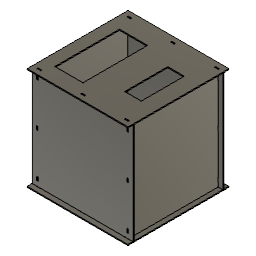
MA GreenForge Greenhouse v21 (Autodesk Fusion 360 design; units mm, degrees)
Autodesk Fusion 360 part; units mm, degrees
sketch "Sketch1" plane through (0, 0, 0) normal (0, 0, 1) x (1, 0, 0)
  line L0 (-377.9, 133.9) -> (-377.9, 137.4)
  line L1 (-631.7, 137.4) -> (-631.7, 133.9)
  line L2 (-631.7, 133.9) -> (-642.2, 133.9)
  line L3 (-642.2, -133.9) -> (-631.7, -133.9)
  line L4 (-367.4, 137.4) -> (-367.4, 133.9)
  line L5 (-642.2, 137.4) -> (-631.7, 137.4)
  line L6 (-657.2, 152.4) -> (-352.4, 152.4)
  line L7 (-352.4, -152.4) -> (-657.2, 152.4) construction
  line L8 (-352.4, 152.4) -> (-352.4, -152.4)
  line L9 (-657.2, -152.4) -> (-657.2, 152.4)
  line L10 (-657.2, -152.4) -> (-352.4, 152.4) construction
  line L11 (-642.2, -137.4) -> (-642.2, -133.9)
  line L12 (-367.4, -137.4) -> (-377.9, -137.4)
  line L13 (-352.4, -152.4) -> (-657.2, -152.4)
  line L14 (-377.9, -133.9) -> (-367.4, -133.9)
  line L15 (-631.7, -137.4) -> (-642.2, -137.4)
  line L16 (-377.9, -137.4) -> (-377.9, -133.9)
  line L17 (-367.4, -133.9) -> (-367.4, -137.4)
  line L18 (-631.7, -133.9) -> (-631.7, -137.4)
  line L19 (-642.2, 133.9) -> (-642.2, 137.4)
  line L20 (-377.9, 137.4) -> (-367.4, 137.4)
  line L21 (-367.4, 133.9) -> (-377.9, 133.9)
  line L22 (-499.55, 133.9) -> (-510.05, 133.9)
  line L23 (-510.05, 133.9) -> (-510.05, 137.4)
  line L24 (-510.05, 137.4) -> (-499.55, 137.4)
  line L25 (-499.55, 137.4) -> (-499.55, 133.9)
  line L26 (-499.55, 133.9) -> (-510.05, 137.4) construction
  line L27 (-510.05, 133.9) -> (-499.55, 137.4) construction
  line L28 (-499.55, -137.4) -> (-510.05, -137.4)
  line L29 (-510.05, -137.4) -> (-510.05, -133.9)
  line L30 (-510.05, -133.9) -> (-499.55, -133.9)
  line L31 (-499.55, -133.9) -> (-499.55, -137.4)
  line L32 (-499.55, -137.4) -> (-510.05, -133.9) construction
  line L33 (-510.05, -137.4) -> (-499.55, -133.9) construction
  line L34 (-126.9, 137.4) -> (-126.9, 133.9)
  line L35 (126.9, 133.9) -> (126.9, 137.4)
  line L36 (-137.4, 133.9) -> (-137.4, 137.4)
  line L37 (137.4, -133.9) -> (137.4, -137.4)
  line L38 (-5.25, 137.4) -> (5.25, 137.4)
  line L39 (5.25, -137.4) -> (-5.25, -137.4)
  line L40 (152.4, 152.4) -> (152.4, -152.4)
  line L41 (126.9, -137.4) -> (126.9, -133.9)
  line L42 (-152.4, -152.4) -> (-152.4, 152.4)
  line L43 (-5.25, -133.9) -> (5.25, -133.9)
  line L44 (-5.25, 133.9) -> (-5.25, 137.4)
  line L45 (-5.25, 133.9) -> (5.25, 137.4) construction
  line L46 (-137.4, 137.4) -> (-126.9, 137.4)
  line L47 (5.25, 133.9) -> (-5.25, 133.9)
  line L48 (126.9, 137.4) -> (137.4, 137.4)
  line L49 (152.4, -152.4) -> (-152.4, 152.4) construction
  line L50 (5.25, 133.9) -> (-5.25, 137.4) construction
  line L51 (-5.25, -137.4) -> (-5.25, -133.9)
  line L52 (-126.9, -133.9) -> (-126.9, -137.4)
  line L53 (137.4, 133.9) -> (126.9, 133.9)
  line L54 (152.4, -152.4) -> (-152.4, -152.4)
  line L55 (5.25, -137.4) -> (-5.25, -133.9) construction
  line L56 (5.25, -133.9) -> (5.25, -137.4)
  line L57 (137.4, -137.4) -> (126.9, -137.4)
  line L58 (5.25, 137.4) -> (5.25, 133.9)
  line L59 (126.9, -133.9) -> (137.4, -133.9)
  line L60 (-152.4, 152.4) -> (152.4, 152.4)
  line L61 (-152.4, -152.4) -> (152.4, 152.4) construction
  line L62 (-5.25, -137.4) -> (5.25, -133.9) construction
  line L63 (-126.9, 133.9) -> (-137.4, 133.9)
  line L64 (-126.9, -137.4) -> (-137.4, -137.4)
  line L65 (137.4, 137.4) -> (137.4, 133.9)
  line L66 (-137.4, -133.9) -> (-126.9, -133.9)
  line L67 (-137.4, -137.4) -> (-137.4, -133.9)
  line L68 (137.4, 349.4) -> (127.4, 352.4) construction
  line L69 (137.4, 352.4) -> (137.4, 349.4)
  line L70 (4.75, 352.4) -> (127.4, 352.4)
  line L71 (-5.25, 349.4) -> (4.75, 352.4) construction
  line L72 (-137.4, 349.4) -> (-137.4, 352.4)
  line L73 (-5.25, 349.4) -> (-5.25, 352.4)
  line L74 (-152.4, 352.4) -> (-137.4, 352.4)
  line L75 (-137.4, 349.4) -> (-127.4, 352.4) construction
  line L76 (-127.4, 349.4) -> (-137.4, 352.4) construction
  line L77 (137.4, 352.4) -> (152.4, 352.4)
  line L78 (127.4, 349.4) -> (127.4, 352.4)
  line L79 (127.4, 349.4) -> (137.4, 352.4) construction
  line L80 (4.75, 349.4) -> (-5.25, 352.4) construction
  line L81 (137.4, 349.4) -> (127.4, 349.4)
  line L82 (152.4, 352.4) -> (152.4, 621.2)
  line L83 (-127.4, 352.4) -> (-5.25, 352.4)
  line L84 (4.75, 352.4) -> (4.75, 349.4)
  line L85 (-5.25, 621.2) -> (4.75, 624.2) construction
  line L86 (4.75, 621.2) -> (-5.25, 624.2) construction
  line L87 (127.4006, 621.2) -> (127.4006, 624.2)
  line L88 (127.4006, 624.2) -> (137.4, 624.3068)
  line L89 (137.4, 624.3068) -> (137.4, 621.2)
  line L90 (-137.4, 621.2) -> (-152.4, 621.2)
  line L91 (-5.25, 624.2) -> (4.75, 624.2)
  line L92 (-127.4, 624.2) -> (-127.4, 621.2)
  line L93 (-5.25, 621.2) -> (-5.25, 624.2)
  line L94 (4.75, 624.2) -> (4.75, 621.2)
  line L95 (-137.4, 621.2) -> (-127.4, 624.2) construction
  line L96 (-137.4, 624.2) -> (-127.4, 624.2)
  line L97 (152.4, 621.2) -> (137.4, 621.2)
  line L98 (-5.25, 621.2) -> (-127.4, 621.2)
  line L99 (127.4006, 621.2) -> (4.75, 621.2)
  line L100 (-127.4, 621.2) -> (-137.4, 624.2) construction
  line L101 (-137.4, 621.2) -> (-137.4, 624.2)
  line L102 (-152.4, 621.2) -> (152.4, 352.4) construction
  line L103 (-152.4, 621.2) -> (-152.4, 352.4)
  line L104 (4.75, 349.4) -> (-5.25, 349.4)
  line L105 (-127.4, 349.4) -> (-137.4, 349.4)
  line L106 (127.4006, 621.2) -> (137.4, 624.3068) construction
  line L107 (137.4, 621.2) -> (127.4006, 624.2) construction
  line L108 (152.4, 621.2) -> (-152.4, 352.4) construction
  line L109 (-127.4, 352.4) -> (-127.4, 349.4)
  line L110 (-620.875, 90) -> (-535.875, 90)
  line L111 (-535.875, 90) -> (-535.875, -105)
  line L112 (-535.875, -105) -> (-620.875, -105)
  line L113 (-620.875, -105) -> (-620.875, 90)
  line L114 (-400, 65) -> (-450, 65)
  line L115 (-450, 65) -> (-450, -65)
  line L116 (-450, -65) -> (-400, -65)
  line L117 (-400, -65) -> (-400, 65)
  line L118 (-458.1406, 349.4) -> (-468.1406, 349.4)
  line L119 (-335.4884, 624.2) -> (-325.4906, 623.9923)
  line L120 (-468.1406, 624.2) -> (-468.1406, 621.2)
  line L121 (-325.4906, 352.4) -> (-310.4906, 352.4)
  line L122 (-615.2906, 621.2) -> (-310.4906, 352.4) construction
  line L123 (-335.4906, 349.4) -> (-325.4906, 352.4) construction
  line L124 (-458.1406, 352.4) -> (-335.4906, 352.4)
  line L125 (-458.1406, 621.2) -> (-458.1406, 624.2)
  line L126 (-310.4906, 621.2) -> (-615.2906, 352.4) construction
  line L127 (-325.4906, 349.4) -> (-335.4906, 349.4)
  line L128 (-335.4884, 621.2) -> (-458.1406, 621.2)
  line L129 (-600.2906, 621.2) -> (-600.2906, 624.2)
  line L130 (-468.1406, 349.4) -> (-468.1406, 352.4)
  line L131 (-335.4884, 621.2) -> (-325.4906, 623.9923) construction
  line L132 (-615.2906, 352.4) -> (-600.2906, 352.4)
  line L133 (-590.2906, 352.4) -> (-468.1406, 352.4)
  line L134 (-590.2906, 624.2) -> (-590.2906, 621.2)
  line L135 (-600.2906, 349.4) -> (-590.2906, 352.4) construction
  line L136 (-590.2906, 621.2) -> (-600.2906, 624.2) construction
  line L137 (-590.2906, 349.4) -> (-600.2906, 352.4) construction
  line L138 (-468.1406, 621.2) -> (-590.2906, 621.2)
  line L139 (-590.2906, 352.4) -> (-590.2906, 349.4)
  line L140 (-600.2906, 349.4) -> (-600.2906, 352.4)
  line L141 (-325.4906, 623.9923) -> (-325.4906, 621.2)
  line L142 (-335.4884, 621.2) -> (-335.4884, 624.2)
  line L143 (-458.1406, 352.4) -> (-458.1406, 349.4)
  line L144 (-335.4906, 349.4) -> (-335.4906, 352.4)
  line L145 (-458.1406, 621.2) -> (-468.1406, 624.2) construction
  line L146 (-600.2906, 621.2) -> (-615.2906, 621.2)
  line L147 (-600.2906, 624.2) -> (-590.2906, 624.2)
  line L148 (-590.2906, 349.4) -> (-600.2906, 349.4)
  line L149 (-615.2906, 621.2) -> (-615.2906, 352.4)
  line L150 (-600.2906, 621.2) -> (-590.2906, 624.2) construction
  line L151 (-458.1406, 624.2) -> (-468.1406, 624.2)
  line L152 (-468.1406, 349.4) -> (-458.1406, 352.4) construction
  line L153 (-310.4906, 352.4) -> (-310.4906, 621.2)
  line L154 (-310.4906, 621.2) -> (-325.4906, 621.2)
  line L155 (-325.4906, 621.2) -> (-335.4884, 624.2) construction
  line L156 (-458.1406, 349.4) -> (-468.1406, 352.4) construction
  line L157 (-325.4906, 349.4) -> (-335.4906, 352.4) construction
  line L158 (-325.4906, 352.4) -> (-325.4906, 349.4)
  line L159 (-468.1406, 621.2) -> (-458.1406, 624.2) construction
  line L160 (377.4, -147.708) -> (377.4, -150.708)
  line L161 (632.2, 160.092) -> (642.2, 160.092)
  line L162 (367.4, 157.092) -> (377.4, 160.092) construction
  line L163 (632.2, 157.092) -> (632.2, 160.092)
  line L164 (499.55, 160.092) -> (509.55, 160.092)
  line L165 (642.2, 160.092) -> (642.2, 157.092)
  line L166 (499.55, 157.092) -> (499.55, 160.092)
  line L167 (509.55, 160.092) -> (509.55, 157.092)
  line L168 (367.4, 157.092) -> (352.4, 157.092)
  line L169 (501.587, -147.708) -> (632.2, -147.708)
  line L170 (367.4, 157.092) -> (367.4, 160.092)
  line L171 (499.55, 157.092) -> (377.4, 157.092)
  line L172 (367.4, 160.092) -> (377.4, 160.092)
  line L173 (377.4, 160.092) -> (377.4, 157.092)
  line L174 (632.2, 157.092) -> (642.2, 160.092) construction
  line L175 (642.2, 157.092) -> (632.2, 160.092) construction
  line L176 (352.4, -147.708) -> (367.4, -147.708)
  line L177 (642.2, -147.708) -> (642.2, -150.708)
  line L178 (367.4, -150.708) -> (377.4, -147.708) construction
  line L179 (642.2, -150.708) -> (632.2, -150.708)
  line L180 (509.55, -148.7712) -> (499.55, -148.7712)
  line L181 (509.55, -143.5517) -> (509.55, -148.7712)
  line L182 (499.55, -148.7712) -> (509.55, -143.5517) construction
  line L183 (632.2, -150.708) -> (642.2, -147.708) construction
  line L184 (642.2, -150.708) -> (632.2, -147.708) construction
  line L185 (377.4, -150.708) -> (367.4, -150.708)
  line L186 (632.2, -150.708) -> (632.2, -147.708)
  line L187 (509.55, -148.7712) -> (499.55, -145.7712) construction
  line L188 (642.2, -147.708) -> (657.2, -147.708)
  line L189 (377.4, -147.708) -> (506.006, -147.708)
  line L190 (499.55, -148.7712) -> (499.55, -145.7712)
  line L191 (657.2, 157.092) -> (352.4, -147.708) construction
  line L192 (377.4, -150.708) -> (367.4, -147.708) construction
  line L193 (367.4, -150.708) -> (367.4, -147.708)
  line L194 (657.2, -147.708) -> (657.2, 157.092)
  line L195 (499.55, 157.092) -> (509.55, 160.092) construction
  line L196 (377.4, 157.092) -> (367.4, 160.092) construction
  line L197 (509.55, 157.092) -> (499.55, 160.092) construction
  line L198 (657.2, 157.092) -> (642.2, 157.092)
  line L199 (632.2, 157.092) -> (509.55, 157.092)
  line L200 (352.4, 157.092) -> (657.2, -147.708) construction
  line L201 (352.4, 157.092) -> (352.4, -147.708)
  line L202 (370.9, -132.708) -> (367.4, -132.708)
  line L203 (367.4, -132.708) -> (367.4, -122.208)
  line L204 (367.4, -122.208) -> (370.9, -122.208)
  line L205 (370.9, -122.208) -> (370.9, -132.708)
  line L206 (370.9, -132.708) -> (367.4, -122.208) construction
  line L207 (367.4, -132.708) -> (370.9, -122.208) construction
  line L208 (369.15, -0.558) -> (365.65, -0.558)
  line L209 (365.65, -0.558) -> (365.65, 9.942)
  line L210 (365.65, 9.942) -> (369.15, 9.942)
  line L211 (369.15, 9.942) -> (369.15, -0.558)
  line L212 (369.15, -0.558) -> (365.65, 9.942) construction
  line L213 (365.65, -0.558) -> (369.15, 9.942) construction
  line L214 (370.9, 131.592) -> (367.4, 131.592)
  line L215 (367.4, 131.592) -> (367.4, 142.092)
  line L216 (367.4, 142.092) -> (370.9, 142.092)
  line L217 (370.9, 142.092) -> (370.9, 131.592)
  line L218 (370.9, 131.592) -> (367.4, 142.092) construction
  line L219 (367.4, 131.592) -> (370.9, 142.092) construction
  line L220 (638.7, 131.592) -> (642.2, 131.592)
  line L221 (642.2, 131.592) -> (642.2, 142.092)
  line L222 (642.2, 142.092) -> (638.7, 142.092)
  line L223 (638.7, 142.092) -> (638.7, 131.592)
  line L224 (638.7, 131.592) -> (642.2, 142.092) construction
  line L225 (642.2, 131.592) -> (638.7, 142.092) construction
  line L226 (638.7, -0.558) -> (642.2, -0.558)
  line L227 (642.2, -0.558) -> (642.2, 9.942)
  line L228 (642.2, 9.942) -> (638.7, 9.942)
  line L229 (638.7, 9.942) -> (638.7, -0.558)
  line L230 (638.7, -0.558) -> (642.2, 9.942) construction
  line L231 (642.2, -0.558) -> (638.7, 9.942) construction
  line L232 (642.2, -132.708) -> (638.7, -132.708)
  line L233 (638.7, -132.708) -> (638.7, -122.208)
  line L234 (638.7, -122.208) -> (642.2, -122.208)
  line L235 (642.2, -122.208) -> (642.2, -132.708)
  line L236 (642.2, -132.708) -> (638.7, -122.208) construction
  line L237 (638.7, -132.708) -> (642.2, -122.208) construction
  line L238 (657.2, 661.892) -> (642.2, 661.892)
  line L239 (638.7, 504.242) -> (642.2, 504.242)
  line L240 (367.4, 661.892) -> (377.4, 664.892) construction
  line L241 (642.2, 372.092) -> (638.7, 382.592) construction
  line L242 (365.65, 514.742) -> (369.15, 514.742)
  line L243 (370.9, 636.392) -> (367.4, 646.892) construction
  line L244 (632.2, 354.092) -> (632.2, 357.092)
  line L245 (499.55, 661.892) -> (509.55, 664.892) construction
  line L246 (370.9, 636.392) -> (367.4, 636.392)
  line L247 (499.55, 661.892) -> (377.4, 661.892)
  line L248 (367.4, 661.892) -> (352.4, 661.892)
  line L249 (642.2, 636.392) -> (642.2, 646.892)
  line L250 (377.4, 664.892) -> (377.4, 661.892)
  line L251 (638.7, 372.092) -> (638.7, 382.592)
  line L252 (642.2, 354.092) -> (632.2, 357.092) construction
  line L253 (367.4, 636.392) -> (370.9, 646.892) construction
  line L254 (509.55, 357.092) -> (509.55, 354.092)
  line L255 (499.55, 354.092) -> (499.55, 357.092)
  line L256 (370.9, 646.892) -> (370.9, 636.392)
  line L257 (369.15, 504.242) -> (365.65, 504.242)
  line L258 (638.7, 372.092) -> (642.2, 382.592) construction
  line L259 (377.4, 661.892) -> (367.4, 664.892) construction
  line L260 (367.4, 372.092) -> (367.4, 382.592)
  line L261 (642.2, 357.092) -> (642.2, 354.092)
  line L262 (367.4, 661.892) -> (367.4, 664.892)
  line L263 (642.2, 382.592) -> (642.2, 372.092)
  line L264 (377.4, 354.092) -> (367.4, 357.092) construction
  line L265 (509.55, 354.092) -> (499.55, 357.092) construction
  line L266 (367.4, 354.092) -> (377.4, 357.092) construction
  line L267 (499.55, 354.092) -> (509.55, 357.092) construction
  line L268 (632.2, 354.092) -> (642.2, 357.092) construction
  line L269 (367.4, 646.892) -> (370.9, 646.892)
  line L270 (377.4, 357.092) -> (377.4, 354.092)
  line L271 (370.9, 372.092) -> (367.4, 382.592) construction
  line L272 (509.55, 354.092) -> (499.55, 354.092)
  line L273 (509.55, 357.092) -> (632.2, 357.092)
  line L274 (370.9, 382.592) -> (370.9, 372.092)
  line L275 (642.2, 354.092) -> (632.2, 354.092)
  line L276 (642.2, 664.892) -> (642.2, 661.892)
  line L277 (632.2, 661.892) -> (642.2, 664.892) construction
  line L278 (367.4, 354.092) -> (367.4, 357.092)
  line L279 (370.9, 372.092) -> (367.4, 372.092)
  line L280 (632.2, 661.892) -> (509.55, 661.892)
  line L281 (377.4, 354.092) -> (367.4, 354.092)
  line L282 (367.4, 382.592) -> (370.9, 382.592)
  line L283 (352.4, 357.092) -> (367.4, 357.092)
  line L284 (367.4, 372.092) -> (370.9, 382.592) construction
  line L285 (657.2, 661.892) -> (352.4, 357.092) construction
  line L286 (638.7, 636.392) -> (642.2, 636.392)
  line L287 (499.55, 664.892) -> (509.55, 664.892)
  line L288 (642.2, 636.392) -> (638.7, 646.892) construction
  line L289 (509.55, 661.892) -> (499.55, 664.892) construction
  line L290 (642.2, 514.742) -> (638.7, 514.742)
  line L291 (365.65, 504.242) -> (365.65, 514.742)
  line L292 (352.4, 661.892) -> (352.4, 357.092)
  line L293 (369.15, 514.742) -> (369.15, 504.242)
  line L294 (352.4, 661.892) -> (657.2, 357.092) construction
  line L295 (632.2, 664.892) -> (642.2, 664.892)
  line L296 (499.55, 661.892) -> (499.55, 664.892)
  line L297 (642.2, 646.892) -> (638.7, 646.892)
  line L298 (632.2, 661.892) -> (632.2, 664.892)
  line L299 (638.7, 636.392) -> (642.2, 646.892) construction
  line L300 (367.4, 636.392) -> (367.4, 646.892)
  line L301 (367.4, 664.892) -> (377.4, 664.892)
  line L302 (642.2, 661.892) -> (632.2, 664.892) construction
  line L303 (638.7, 382.592) -> (642.2, 382.592)
  line L304 (642.2, 357.092) -> (657.2, 357.092)
  line L305 (377.4, 357.092) -> (499.55, 357.092)
  line L306 (642.2, 372.092) -> (638.7, 372.092)
  line L307 (642.2, 504.242) -> (638.7, 514.742) construction
  line L308 (369.15, 504.242) -> (365.65, 514.742) construction
  line L309 (657.2, 357.092) -> (657.2, 661.892)
  line L310 (638.7, 514.742) -> (638.7, 504.242)
  line L311 (638.7, 504.242) -> (642.2, 514.742) construction
  line L312 (642.2, 504.242) -> (642.2, 514.742)
  line L313 (638.7, 646.892) -> (638.7, 636.392)
  line L314 (509.55, 664.892) -> (509.55, 661.892)
  line L315 (365.65, 504.242) -> (369.15, 514.742) construction
  point P0 (-504.8, 0)
  point P1 (-504.8, 135.65)
  point P2 (-504.8, -135.65)
  point P3 (0, 135.65)
  point P4 (0, -135.65)
  point P5 (-132.4, 622.7)
  point P6 (-0.25, 622.7)
  point P7 (0, 486.8)
  point P8 (-132.4, 350.9)
  point P9 (132.4, 350.9)
  point P10 (132.3129, 622.7262)
  point P11 (-595.2906, 350.9)
  point P12 (-330.4906, 350.9)
  point P13 (-595.2906, 622.7)
  point P14 (-463.1406, 622.7)
  point P15 (-330.3102, 622.6462)
  point P16 (-462.8906, 486.8)
  point P17 (372.4, -149.208)
  point P18 (504.8, 4.692)
  point P19 (372.4, 158.592)
  point P20 (504.55, 158.592)
  point P21 (637.2, -149.208)
  point P22 (637.2, 158.592)
  point P23 (369.15, -127.458)
  point P24 (367.4, 4.692)
  point P25 (369.15, 136.842)
  point P26 (640.45, 136.842)
  point P27 (640.45, 4.692)
  point P28 (640.45, -127.458)
  point P29 (640.45, 509.492)
  point P30 (640.45, 641.642)
  point P31 (367.4, 509.492)
  point P32 (640.45, 377.342)
  point P33 (369.15, 377.342)
  point P34 (372.4, 355.592)
  point P35 (504.8, 509.492)
  point P36 (372.4, 663.392)
  point P37 (504.55, 663.392)
  point P38 (637.2, 355.592)
  point P39 (637.2, 663.392)
  point P40 (369.15, 641.642)
  dimension "d45" = 304.8
  dimension "d46" = 304.8
  dimension "d47" = 10.5
  dimension "d48" = 3.5
  dimension "d49" = 15
  dimension "d50" = 15
  dimension "d51" = 15
  dimension "d52" = 15
  dimension "d53" = 3.5
  dimension "d54" = 15
  dimension "d55" = 15
  dimension "d56" = 15
  dimension "d57" = 15
  dimension "d96" = 147.15
  dimension "d97" = 15
  dimension "d99" = 147.15
  dimension "d100" = 304.8
  dimension "d101" = 304.8
  dimension "d102" = 10.5
  dimension "d103" = 3.5
  dimension "d104" = 15
  dimension "d105" = 15
  dimension "d106" = 15
  dimension "d107" = 15
  dimension "d108" = 3.5
  dimension "d109" = 15
  dimension "d110" = 15
  dimension "d111" = 15
  dimension "d112" = 15
  dimension "d113" = 147.15
  dimension "d114" = 15
  dimension "d116" = 147.15
  dimension "d117" = 200
  dimension "d163" = 15
  dimension "d164" = 15
  dimension "d260" = 268.8
  dimension "d261" = 304.8
  dimension "d262" = 10
  dimension "d263" = 3
  dimension "d264" = 15
  dimension "d265" = 10
  dimension "d266" = 10
  dimension "d267" = 15
  dimension "d268" = 15
  dimension "d269" = 15
  dimension "d281" = 147.15
  dimension "d282" = 147.15
  dimension "d286" = 200
  dimension "d336" = 85
  dimension "d337" = 195
  dimension "d338" = 31.075
  dimension "d340" = 47.6
  dimension "d341" = 130
  dimension "d342" = 87.4
  dimension "d343" = 50
  dimension "d356" = 3
  dimension "d357" = 90
  dimension "d358" = 3
  dimension "d359" = 268.8
  dimension "d360" = 304.8
  dimension "d361" = 10
  dimension "d362" = 3
  dimension "d363" = 15
  dimension "d364" = 10
  dimension "d365" = 10
  dimension "d366" = 15
  dimension "d367" = 15
  dimension "d368" = 15
  dimension "d370" = 147.15
  dimension "d371" = 3
  dimension "d372" = 90
  dimension "d373" = 3
  dimension "d374" = 304.8
  dimension "d375" = 304.8
  dimension "d376" = 10
  dimension "d377" = 3
  dimension "d378" = 15
  dimension "d379" = 10
  dimension "d380" = 10
  dimension "d381" = 15
  dimension "d382" = 15
  dimension "d383" = 15
  dimension "d390" = 147.15
  dimension "d391" = 147.15
  dimension "d410" = 200
  dimension "d429" = 15
  dimension "d430" = 15
  dimension "d431" = 3.5
  dimension "d432" = 10.5
  dimension "d433" = 15
  dimension "d434" = 147.15
  dimension "d435" = 15
  dimension "d436" = 15
  dimension "d437" = 15
  dimension "d438" = 15
  dimension "d439" = 3.5
  dimension "d440" = 15
  dimension "d441" = 15
  dimension "d442" = 15
  dimension "d443" = 147.15
  dimension "d473" = 304.8
  dimension "d474" = 304.8
  dimension "d475" = 10
  dimension "d476" = 3
  dimension "d477" = 15
  dimension "d478" = 10
  dimension "d479" = 10
  dimension "d480" = 15
  dimension "d481" = 15
  dimension "d482" = 15
  dimension "d483" = 147.15
  dimension "d484" = 147.15
  dimension "d485" = 15
  dimension "d486" = 15
  dimension "d487" = 3.5
  dimension "d488" = 10.5
  dimension "d489" = 15
  dimension "d490" = 147.15
  dimension "d491" = 15
  dimension "d492" = 15
  dimension "d493" = 15
  dimension "d494" = 15
  dimension "d495" = 3.5
  dimension "d496" = 15
  dimension "d497" = 15
  dimension "d498" = 15
  dimension "d499" = 147.15
  dimension "d500" = 200
  dimension "d501" = 200
  dimension "d522" = 147.15
  dimension "d535" = 3
  dimension "d537" = 90
  dimension "d538" = 90
  dimension "d539" = 90
  dimension "d540" = 90
  dimension "d541" = 90
  constraint horizontal L13
  constraint perpendicular L9 L13
  constraint parallel L6 L13
  constraint parallel L8 L9
  constraint coincident P0 L7
  constraint coincident P0 L10
  constraint horizontal L5
  constraint vertical L1
  constraint horizontal L2
  constraint vertical L19
  constraint horizontal L20
  constraint vertical L4
  constraint horizontal L21
  constraint vertical L0
  constraint horizontal L3
  constraint vertical L18
  constraint horizontal L15
  constraint vertical L11
  constraint horizontal L14
  constraint vertical L17
  constraint horizontal L12
  constraint vertical L16
  constraint equal L2 L20
  constraint equal L2 L3
  constraint equal L3 L14
  constraint equal L0 L1
  constraint equal L16 L18
  constraint horizontal L22
  constraint perpendicular L22 L23
  constraint parallel L22 L24
  constraint parallel L23 L25
  constraint coincident L26 P1
  constraint coincident L27 P1
  constraint equal L19 L23
  constraint equal L5 L24
  constraint horizontal L28
  constraint perpendicular L28 L29
  constraint parallel L28 L30
  constraint parallel L29 L31
  constraint coincident L32 P2
  constraint coincident L33 P2
  constraint equal L11 L29
  constraint equal L3 L30
  constraint horizontal L54
  constraint perpendicular L42 L54
  constraint parallel L54 L60
  constraint parallel L40 L42
  constraint coincident origin L49
  constraint coincident origin L61
  constraint horizontal L46
  constraint vertical L34
  constraint horizontal L63
  constraint vertical L36
  constraint horizontal L48
  constraint vertical L65
  constraint horizontal L53
  constraint vertical L35
  constraint horizontal L66
  constraint vertical L52
  constraint horizontal L64
  constraint vertical L67
  constraint horizontal L59
  constraint vertical L37
  constraint horizontal L57
  constraint vertical L41
  constraint equal L48 L63
  constraint equal L63 L66
  constraint equal L59 L66
  constraint equal L34 L35
  constraint equal L41 L52
  constraint horizontal L47
  constraint perpendicular L44 L47
  constraint parallel L38 L47
  constraint parallel L44 L58
  constraint coincident P3 L50
  constraint coincident P3 L45
  constraint equal L36 L44
  constraint equal L38 L46
  constraint horizontal L39
  constraint perpendicular L39 L51
  constraint parallel L39 L43
  constraint parallel L51 L56
  constraint coincident P4 L55
  constraint coincident P4 L62
  constraint equal L51 L67
  constraint equal L43 L66
  constraint collinear L6 L60
  constraint horizontal L97
  constraint perpendicular L97 L103
  constraint parallel L74 L97
  constraint parallel L82 L103
  constraint coincident P7 L108
  constraint coincident P7 L102
  constraint parallel L92 L101
  constraint coincident P5 L100
  constraint coincident P5 L95
  constraint parallel L87 L89
  constraint coincident P10 L107
  constraint coincident P10 L106
  constraint horizontal L105
  constraint perpendicular L72 L105
  constraint parallel L72 L109
  constraint coincident P8 L76
  constraint coincident P8 L75
  constraint horizontal L81
  constraint perpendicular L78 L81
  constraint parallel L69 L78
  constraint coincident P9 L68
  constraint coincident P9 L79
  constraint equal L72 L78
  constraint equal L78 L87
  constraint equal L87 L101
  constraint equal L88 L96
  constraint collinear L90 L97
  constraint collinear L97 L99
  constraint collinear L74 L83
  constraint collinear L77 L83
  constraint parallel L93 L94
  constraint coincident P6 L86
  constraint coincident P6 L85
  constraint equal L92 L93
  constraint equal L91 L96
  constraint horizontal L104
  constraint perpendicular L73 L104
  constraint parallel L73 L84
  constraint equal L72 L73
  constraint equal L104 L105
  constraint coincident L73.end L80
  constraint coincident L70.start L71
  constraint collinear L70 L83
  constraint collinear L98 L99
  constraint collinear L40 L82
  constraint horizontal L110
  constraint vertical L111
  constraint horizontal L112
  constraint vertical L113
  constraint horizontal L114
  constraint vertical L115
  constraint horizontal L116
  constraint vertical L117
  constraint coincident L73.end L80.end
  constraint horizontal L154
  constraint perpendicular L149 L154
  constraint parallel L132 L154
  constraint parallel L149 L153
  constraint coincident P16 L126
  constraint coincident P16 L122
  constraint parallel L129 L134
  constraint coincident P13 L136
  constraint coincident P13 L150
  constraint parallel L141 L142
  constraint coincident P15 L155
  constraint coincident P15 L131
  constraint horizontal L148
  constraint perpendicular L140 L148
  constraint parallel L139 L140
  constraint coincident P11 L137
  constraint coincident P11 L135
  constraint horizontal L127
  constraint perpendicular L127 L144
  constraint parallel L144 L158
  constraint coincident P12 L157
  constraint coincident P12 L123
  constraint equal L140 L144
  constraint equal L142 L144
  constraint equal L129 L142
  constraint equal L119 L147
  constraint collinear L146 L154
  constraint collinear L128 L154
  constraint collinear L132 L133
  constraint collinear L121 L133
  constraint parallel L120 L125
  constraint coincident P14 L159
  constraint coincident P14 L145
  constraint equal L125 L134
  constraint equal L147 L151
  constraint horizontal L118
  constraint perpendicular L118 L130
  constraint parallel L130 L143
  constraint equal L130 L140
  constraint equal L118 L148
  constraint coincident L130.end L156
  constraint coincident L124.start L152
  constraint collinear L124 L133
  constraint coincident L125.start L145
  constraint collinear L128 L138
  constraint coincident L130.end L133.end
  constraint coincident L128.end L125
  constraint horizontal L198
  constraint perpendicular L198 L201
  constraint parallel L176 L198
  constraint parallel L194 L201
  constraint coincident P18 L191
  constraint coincident P18 L200
  constraint parallel L170 L173
  constraint coincident P19 L196
  constraint coincident P19 L162
  constraint parallel L163 L165
  constraint coincident P22 L175
  constraint coincident P22 L174
  constraint horizontal L185
  constraint perpendicular L185 L193
  constraint parallel L160 L193
  constraint coincident P17 L192
  constraint coincident P17 L178
  constraint horizontal L179
  constraint perpendicular L179 L186
  constraint parallel L177 L186
  constraint coincident P21 L184
  constraint coincident P21 L183
  constraint equal L186 L193
  constraint equal L163 L186
  constraint equal L163 L170
  constraint equal L161 L172
  constraint collinear L168 L198
  constraint collinear L198 L199
  constraint collinear L176 L189
  constraint collinear L188 L189
  constraint parallel L166 L167
  constraint coincident P20 L197
  constraint coincident P20 L195
  constraint equal L166 L173
  constraint equal L164 L172
  constraint horizontal L180
  constraint perpendicular L180 L190
  constraint parallel L181 L190
  constraint equal L190 L193
  constraint equal L180 L185
  constraint coincident L189.end L187
  constraint coincident L169.start L182
  constraint collinear L169 L189
  constraint coincident L167.end L197
  constraint coincident L166.start L195
  constraint collinear L171 L199
  constraint horizontal L202
  constraint perpendicular L202 L203
  constraint parallel L202 L204
  constraint parallel L203 L205
  constraint coincident L206 P23
  constraint coincident L207 P23
  constraint horizontal L208
  constraint perpendicular L208 L209
  constraint parallel L208 L210
  constraint parallel L209 L211
  constraint coincident L212 P24
  constraint coincident L213 P24
  constraint equal L204 L208
  constraint equal L203 L209
  constraint horizontal L214
  constraint perpendicular L214 L215
  constraint parallel L214 L216
  constraint parallel L215 L217
  constraint coincident L218 P25
  constraint coincident L219 P25
  constraint horizontal L220
  constraint perpendicular L220 L221
  constraint parallel L220 L222
  constraint parallel L221 L223
  constraint coincident L224 P26
  constraint coincident L225 P26
  constraint horizontal L226
  constraint perpendicular L226 L227
  constraint parallel L226 L228
  constraint parallel L227 L229
  constraint coincident L230 P27
  constraint coincident L231 P27
  constraint horizontal L232
  constraint perpendicular L232 L233
  constraint parallel L232 L234
  constraint parallel L233 L235
  constraint coincident L236 P28
  constraint coincident L237 P28
  constraint equal L211 L217
  constraint equal L217 L223
  constraint equal L210 L216
  constraint equal L216 L222
  constraint equal L223 L229
  constraint equal L229 L233
  constraint equal L228 L234
  constraint horizontal L238
  constraint perpendicular L238 L292
  constraint parallel L238 L283
  constraint parallel L292 L309
  constraint coincident P35 L285
  constraint coincident P35 L294
  constraint parallel L250 L262
  constraint coincident P36 L259
  constraint coincident P36 L240
  constraint parallel L276 L298
  constraint coincident P39 L302
  constraint coincident P39 L277
  constraint horizontal L281
  constraint perpendicular L278 L281
  constraint parallel L270 L278
  constraint coincident P34 L264
  constraint coincident P34 L266
  constraint horizontal L275
  constraint perpendicular L244 L275
  constraint parallel L244 L261
  constraint coincident P38 L252
  constraint coincident P38 L268
  constraint equal L244 L278
  constraint equal L244 L298
  constraint equal L262 L298
  constraint equal L295 L301
  constraint collinear L238 L248
  constraint collinear L238 L280
  constraint collinear L283 L305
  constraint collinear L304 L305
  constraint parallel L296 L314
  constraint coincident P37 L289
  constraint coincident P37 L245
  constraint equal L250 L296
  constraint equal L287 L301
  constraint horizontal L272
  constraint perpendicular L255 L272
  constraint parallel L254 L255
  constraint equal L255 L278
  constraint equal L272 L281
  constraint coincident L255.end L265
  constraint coincident L254.start L267
  constraint collinear L273 L305
  constraint coincident L280.end L289
  constraint coincident L247.start L245
  constraint collinear L247 L280
  constraint horizontal L279
  constraint perpendicular L260 L279
  constraint parallel L279 L282
  constraint parallel L260 L274
  constraint coincident P33 L271
  constraint coincident P33 L284
  constraint horizontal L257
  constraint perpendicular L257 L291
  constraint parallel L242 L257
  constraint parallel L291 L293
  constraint coincident P31 L308
  constraint coincident P31 L315
  constraint equal L257 L282
  constraint equal L260 L291
  constraint horizontal L246
  constraint perpendicular L246 L300
  constraint parallel L246 L269
  constraint parallel L256 L300
  constraint coincident P40 L243
  constraint coincident P40 L253
  constraint horizontal L286
  constraint perpendicular L249 L286
  constraint parallel L286 L297
  constraint parallel L249 L313
  constraint coincident P30 L299
  constraint coincident P30 L288
  constraint horizontal L239
  constraint perpendicular L239 L312
  constraint parallel L239 L290
  constraint parallel L310 L312
  constraint coincident P29 L311
  constraint coincident P29 L307
  constraint horizontal L306
  constraint perpendicular L251 L306
  constraint parallel L303 L306
  constraint parallel L251 L263
  constraint coincident P32 L241
  constraint coincident P32 L258
  constraint equal L256 L293
  constraint equal L256 L313
  constraint equal L242 L269
  constraint equal L269 L297
  constraint equal L310 L313
  constraint equal L251 L310
  constraint equal L290 L303
  constraint coincident L167.end L197.start
  constraint coincident L166.start L171.start
  constraint coincident L255.end L265.end
  constraint coincident L254.start L267.end
  constraint coincident L245.start L247
  constraint coincident L289.start L280
  measures "d45" distance of L9.start L6.start
  measures "d46" distance of L6.end L6.start
  measures "d47" distance of L5.start L1.start
  measures "d48" distance of L1.end L1.start
  measures "d49" distance of L9 L19
  measures "d50" distance of L5 L6
  measures "d51" distance of L4 L8
  measures "d52" distance of L6 L20
  measures "d53" distance of L3.start L11.start
  measures "d54" distance of L9 L11
  measures "d55" distance of L13 L15
  measures "d56" distance of L12 L13
  measures "d57" distance of L8 L17
  measures "d96" distance of L9 L23
  measures "d97" distance of L6 L24
  measures "d99" distance of L9 L29
  measures "d100" distance of L42.start L42.end
  measures "d101" distance of L40.start L42.end
  measures "d102" distance of L34.start L36.end
  measures "d103" distance of L34.end L34.start
  measures "d104" distance of L36 L42
  measures "d105" distance of L46 L60
  measures "d106" distance of L40 L65
  measures "d107" distance of L48 L60
  measures "d108" distance of L66.start L64.end
  measures "d109" distance of L42 L67
  measures "d110" distance of L54 L64
  measures "d111" distance of L54 L57
  measures "d112" distance of L37 L40
  measures "d113" distance of L42 L44
  measures "d114" distance of L38 L60
  measures "d116" distance of L42 L51
  measures "d117" distance of L8 L42
  measures "d163" distance of L13 L28
  measures "d164" distance of L39 L54
  measures "d260" distance of L90.end L74.start
  measures "d261" distance of L90.end L82.end
  measures "d262" distance of L92.start L96.start
  measures "d263" distance of L90.start L96.start
  measures "d264" distance of L101 L103
  measures "d265" distance of L69.start L68.end
  measures "d266" distance of L72.end L75.end
  measures "d267" distance of L82 L89
  measures "d268" distance of L72 L103
  measures "d269" distance of L69 L82
  measures "d281" distance of L93 L103
  measures "d282" distance of L73 L103
  measures "d286" distance of L60 L70
  measures "d336" distance of L110.start L110.end
  measures "d337" distance of L110.end L111.end
  measures "d338" distance of P0 L111
  measures "d340" distance of L8 L117
  measures "d341" distance of L114.start L116.end
  measures "d342" distance of L6 L114
  measures "d343" distance of L114.start L114.end
  measures "d356" distance of L80.start L70.start
  measures "d357" angle of L91 L94
  measures "d358" distance of L85.end L86.start
  measures "d359" distance of L126.end L122.start
  measures "d360" distance of L126.start L122.start
  measures "d361" distance of L134.start L129.end
  measures "d362" distance of L129.start L129.end
  measures "d363" distance of L129 L149
  measures "d364" distance of L121.start L124.end
  measures "d365" distance of L132.end L133.start
  measures "d366" distance of L141 L153
  measures "d367" distance of L140 L149
  measures "d368" distance of L153 L158
  measures "d370" distance of L130 L149
  measures "d371" distance of L118.start L124.start
  measures "d372" angle of L120 L151
  measures "d373" distance of L120.start L120.end
  measures "d374" distance of L168.end L176.start
  measures "d375" distance of L168.end L191.start
  measures "d376" distance of L162.end L170.end
  measures "d377" distance of L162.start L170.end
  measures "d378" distance of L170 L201
  measures "d379" distance of L169.end L177.start
  measures "d380" distance of L176.end L160.start
  measures "d381" distance of L165 L194
  measures "d382" distance of L193 L201
  measures "d383" distance of L177 L194
  measures "d390" distance of L166 L201
  measures "d391" distance of L190 L201
  measures "d410" distance of L40 L201
  measures "d429" distance of L189 L202
  measures "d430" distance of L201 L203
  measures "d431" distance of L203.end L204.end
  measures "d432" distance of L202.start L204.end
  measures "d433" distance of L201 P24
  measures "d434" distance of L189 L208
  measures "d435" distance of L201 L215
  measures "d436" distance of L171 L216
  measures "d437" distance of L194 L221
  measures "d438" distance of L199 L222
  measures "d439" distance of L227.end L228.end
  measures "d440" distance of L194 L235
  measures "d441" distance of L169 L232
  measures "d442" distance of L194 L227
  measures "d443" distance of L169 L226
  measures "d473" distance of L248.end L283.start
  measures "d474" distance of L248.end L238.start
  measures "d475" distance of L240.end L259.end
  measures "d476" distance of L240.start L259.end
  measures "d477" distance of L262 L292
  measures "d478" distance of L244.end L261.start
  measures "d479" distance of L266.end L264.end
  measures "d480" distance of L276 L309
  measures "d481" distance of L278 L292
  measures "d482" distance of L261 L309
  measures "d483" distance of L292 L296
  measures "d484" distance of L255 L292
  measures "d485" distance of L279 L305
  measures "d486" distance of L260 L292
  measures "d487" distance of L274.start L260.end
  measures "d488" distance of L274.start L271.start
  measures "d489" distance of P31 L292
  measures "d490" distance of L257 L305
  measures "d491" distance of L292 L300
  measures "d492" distance of L247 L269
  measures "d493" distance of L249 L309
  measures "d494" distance of L280 L297
  measures "d495" distance of L290.end L290.start
  measures "d496" distance of L263 L309
  measures "d497" distance of L273 L306
  measures "d498" distance of L309 L312
  measures "d499" distance of L239 L273
  measures "d500" distance of L82 L292
  measures "d501" distance of L199 L273
  measures "d522" distance of L120 L149
  measures "d535" distance of L171.end L162.end
  measures "d537" angle of L164 L167
  measures "d538" angle of L161 L165
  measures "d539" angle of L250 L301
  measures "d540" angle of L287 L314
  measures "d541" angle of L276 L295
extrude "Extrude8" add sketch "Sketch1" along normal blind 3 contours L6 L8 L9 L13 makes body 1
extrude "Extrude9" add sketch "Sketch1" along normal blind 3 separate body contours L118 L119 L120 L121 L124 L125 L127 L128 L129 L130 L132 L133 L134 L138 L139 L140 L141 L142 L143 L144 L146 L147 L148 L149 L151 L153 L154 L158 makes body 2
extrude "Extrude10" add sketch "Sketch1" along normal blind 3 separate body contours L69 L70 L72 L73 L74 L77 L78 L81 L82 L83 L84 L87 L88 L89 L90 L91 L92 L93 L94 L96 L97 L98 L99 L101 L103 L104 L105 L109 makes body 3
extrude "Extrude11" add sketch "Sketch1" along normal blind 3 separate body contours L238 L244 L247 L248 L250 L254 L255 L261 L262 L270 L272 L273 L275 L276 L278 L280 L281 L283 L287 L292 L295 L296 L298 L301 L304 L305 L309 L314 makes body 4
extrude "Extrude12" add sketch "Sketch1" along normal blind 3 separate body contours L160 L161 L163 L164 L165 L166 L167 L168 L169 L170 L171 L172 L173 L176 L177 L179 L185 L186 L188 L189 L193 L194 L198 L199 L201 | L169 L180 L181 L189 L190 makes body 5
extrude "Extrude13" add sketch "Sketch1" along normal blind 3 separate body contours L40 L42 L54 L60 makes body 6
copy_body "Body->Comp7" bodies 1 removing the originals makes body 7 in component "Component"
copy_body "Body->Comp9" bodies 3 removing the originals makes body 8 in component "Component'"
copy_body "Body->Comp10" bodies 4 removing the originals makes body 9 in component "Component''"
copy_body "Body->Comp11" bodies 5 removing the originals makes body 10 in component "Component'''"
copy_body "Body->Comp12" bodies 6 removing the originals makes body 11 in component "Component''''"
copy_body "Body->Comp13" bodies 2 removing the originals makes body 12 in component "Component'''''"
component "Component" placed x (1, 0, 0) y (0, 1, 0) z (0, 0, 1) at (0, 0, 0)
component "Component'" placed x (0, 0, -1) y (0, 1, 0) z (1, 0, 0) at (-370.65, -486.55, -152.9)
component "Component''" placed x (1, 0, 0) y (0, 0, -1) z (0, 1, 0) at (-1009.6, -137.15, 357.092)
component "Component'''" placed x (1, 0, 0) y (0, 0, -1) z (0, 1, 0) at (-1009.6, 134.15, -147.708)
component "Component''''" placed x (1, 0, 0) y (0, 1, 0) z (0, 0, 1) at (-505.3, 0, -307.8)
component "Component'''''" placed x (0, 0, -1) y (0, 1, 0) z (1, 0, 0) at (-643.7, -486.55, -615.7906)
